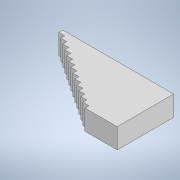
# Autodesk Inventor part: Stairs
Saved by Autodesk Inventor 2021 (Build 250183000, 183)
## iProperties
Created: 2022-07-02
Part Number: Stairs
Material: 一般
Document SubType Name: Modeling
Designer: tazak
Density: 1 g/cm^3
Appearance: 既定
Author: tazak
Autodesk Inventor part; units mm, degrees
ref_plane "YZ Plane" through (0, 0, 0) normal (1, 0, 0) x (0, 1, 0)
ref_plane "XZ Plane" through (0, 0, 0) normal (0, 1, 0) x (-1, 0, 0)
ref_plane "XY Plane" through (0, 0, 0) normal (0, 0, 1) x (1, 0, 0)
sketch "スケッチ1" plane through (0, 0, 0) normal (0, 0, 1) x (1, 0, 0)
  line L0 (5500, 2000) -> (11000, 2000)
  line L1 (11000, 2000) -> (11000, 1000)
  line L2 (11000, 1000) -> (5500, 1000)
  line L3 (5500, 1000) -> (5500, 2000)
  point P0 (0, 0)
  dimension "d13" = 5500
  dimension "d23" = 1000
  dimension "d24" = 5500
  dimension "d28" = 1000
  constraints: 8 end point, 2 parallel, 1 horizontal, 1 perpendicular
  measures "d13" distance of L0.start L0.end
  measures "d23" distance of L2.end L0.start
  measures "d24" distance from line of L3 point (0, 0)
  measures "d28" distance from line of point (0, 0) L2
extrude "押し出し1" add sketch "スケッチ1" along normal blind 2800
sketch "スケッチ6" plane through (5500, 1000, 0) normal (0, -1, 0) x (1, 0, 0)
  line L0 (0, 0) -> (0, 2800) projected
  line L1 (0, 200) -> (300, 200)
  line L2 (300, 200) -> (300, 400)
  line L3 (300, 400) -> (600, 400)
  line L4 (600, 400) -> (600, 600)
  line L5 (600, 600) -> (900, 600)
  line L6 (900, 600) -> (900, 800)
  line L7 (900, 800) -> (1200, 800)
  line L8 (1200, 800) -> (1200, 1000)
  line L9 (1200, 1000) -> (1500, 1000)
  line L10 (1500, 1000) -> (1500, 1200)
  line L11 (1500, 1200) -> (1800, 1200)
  line L12 (0, 0) -> (5500, 0) projected
  line L13 (1800, 1200) -> (1800, 1400)
  line L14 (1800, 1400) -> (2100, 1400)
  line L15 (2100, 1400) -> (2100, 1600)
  line L16 (2100, 1600) -> (2400, 1600)
  line L17 (2400, 1600) -> (2400, 1800)
  line L18 (2400, 1800) -> (2700, 1800)
  line L19 (2700, 1800) -> (2700, 2000)
  line L20 (2700, 2000) -> (3000, 2000)
  line L21 (3000, 2000) -> (3000, 2200)
  line L22 (3000, 2200) -> (3300, 2200)
  line L23 (3300, 2200) -> (3300, 2400)
  line L24 (3300, 2400) -> (3600, 2400)
  line L25 (3600, 2400) -> (3600, 2600)
  line L26 (3600, 2600) -> (3900, 2600)
  line L27 (3900, 2600) -> (3900, 2800)
  line L28 (0, 2800) -> (5500, 2800) projected
  point P0 (-5500, 0)
  dimension "d29" = 300
  dimension "d30" = 300
  dimension "d31" = 300
  dimension "d32" = 300
  dimension "d33" = 300
  dimension "d34" = 300
  dimension "d35" = 200
  dimension "d36" = 200
  dimension "d37" = 200
  dimension "d38" = 200
  dimension "d39" = 200
  dimension "d40" = 200
  dimension "d41" = 300
  dimension "d42" = 300
  dimension "d43" = 300
  dimension "d44" = 300
  dimension "d45" = 300
  dimension "d46" = 300
  dimension "d47" = 200
  dimension "d48" = 200
  dimension "d49" = 200
  dimension "d50" = 200
  dimension "d51" = 200
  dimension "d52" = 200
  dimension "d53" = 300
  dimension "d54" = 200
  constraints: 52 end point, 22 perpendicular, 2 horizontal, 2 point on line, 2 vertical
  measures "d29" distance of L1.start L1.end
  measures "d30" distance of L2.end L3.end
  measures "d31" distance of L4.end L5.end
  measures "d32" distance of L6.end L7.end
  measures "d33" distance of L8.end L9.end
  measures "d34" distance of L10.end L11.end
  measures "d35" distance between parallel lines of L12 L1
  measures "d36" distance of L1.end L2.end
  measures "d37" distance of L3.end L4.end
  measures "d38" distance of L5.end L6.end
  measures "d39" distance of L7.end L8.end
  measures "d40" distance of L9.end L10.end
  measures "d41" distance of L13.end L14.end
  measures "d42" distance of L15.end L16.end
  measures "d43" distance of L17.end L18.end
  measures "d44" distance of L19.end L20.end
  measures "d45" distance of L21.end L22.end
  measures "d46" distance of L23.end L24.end
  measures "d47" distance of L11.end L13.end
  measures "d48" distance of L14.end L15.end
  measures "d49" distance of L16.end L17.end
  measures "d50" distance of L18.end L19.end
  measures "d51" distance of L20.end L21.end
  measures "d52" distance of L22.end L23.end
  measures "d53" distance of L25.end L26.end
  measures "d54" distance of L24.end L25.end
extrude "押し出し6" cut sketch "スケッチ6" against normal through all
